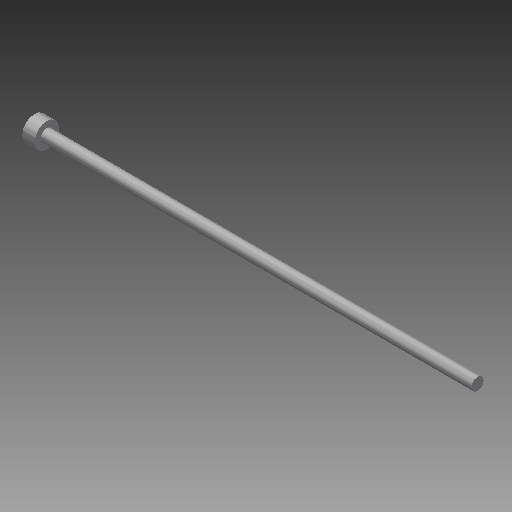
# Autodesk Inventor part: Arbre
Saved by Autodesk Inventor 2017 SP1 (Build 210196100, 196)
## iProperties
Created: 2017-11-26
Part Number: Arbre
Material: Steel
Document SubType Name: Modeling
Designer: Biscuit
Density: 1 g/cm^3
Appearance: Steel
CustomPartVersion: 1
Author: Biscuit
Autodesk Inventor part; units mm, degrees
ref_plane "Plan de départ" through (0, 0, 0) normal (1, 0, 0) x (0, 1, 0)
ref_plane "XZ Plane" through (0, 0, 0) normal (0, 1, 0) x (-1, 0, 0)
ref_plane "XY Plane" through (0, 0, 0) normal (0, 0, 1) x (1, 0, 0)
sketch "Esquisse principale" plane through (0, 0, 0) normal (0, 0, 1) x (1, 0, 0)
  line L0 (0, 0) -> (72, 0)
  line L1 (0, 0) -> (0, 2)
  line L2 (2, 2) -> (2, 1)
  line L3 (0, 2) -> (2, 2)
  line L4 (72, 1) -> (72, 0)
  line L5 (2, 1) -> (72, 1)
  dimension "d3" = 4
  dimension "d4" = 2
  constraints: 12 end point, 4 horizontal, 3 vertical
  measures "d3" diameter of L3 L0
  measures "d4" diameter of L5 L0
revolve "Révolution1" add sketch "Esquisse principale" angle 360 about axis through (0, 0, 0) along (1, 0, 0)
